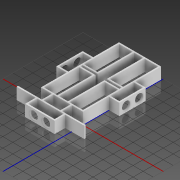
# Autodesk Inventor part: Motorcompartiment
Saved by Autodesk Inventor 2020.2 (Build 242310000, 310)
## iProperties
Created: 2019-12-09
Part Number: Motorcompartiment
Material: Generic
Document SubType Name: Modeling
Designer: Berkant
Density: 1 g/cm^3
Appearance: Default
Author: Berkant
Autodesk Inventor part; units mm, degrees
ref_plane "YZ Plane" through (0, 0, 0) normal (1, 0, 0) x (0, 1, 0)
ref_plane "XZ Plane" through (0, 0, 0) normal (0, 1, 0) x (-1, 0, 0)
ref_plane "XY Plane" through (0, 0, 0) normal (0, 0, 1) x (1, 0, 0)
sketch "Sketch1" plane through (0, 0, 0) normal (0, 1, 0) x (-1, 0, 0)
  line L0 (0, 0) -> (84, 0)
  line L1 (84, 0) -> (84, -156)
  line L2 (0, -156) -> (0, 0)
  line L3 (0, 0) -> (3, 0) construction
  line L4 (3, 0) -> (3, -3) construction
  line L5 (3, -3) -> (0, -3) construction
  line L6 (0, -3) -> (0, 0) construction
  line L7 (84, -153) -> (84, -156) construction
  line L8 (3, -3) -> (30, -3)
  line L9 (30, -3) -> (30, -73)
  line L10 (30, -73) -> (3, -73)
  line L11 (3, -73) -> (3, -3)
  line L12 (78, -153) -> (54, -153)
  line L13 (54, -153) -> (54, -83)
  line L14 (54, -83) -> (81, -83)
  line L15 (81, -83) -> (81, -153)
  line L16 (0, -153) -> (0, -156) construction
  line L17 (84, 0) -> (81, 0) construction
  line L18 (81, 0) -> (81, -3) construction
  line L19 (81, -3) -> (84, -3) construction
  line L20 (84, -3) -> (84, 0) construction
  line L21 (81, -3) -> (54, -3)
  line L22 (54, -3) -> (54, -73)
  line L23 (54, -73) -> (81, -73)
  line L24 (81, -73) -> (81, -3)
  line L25 (6, -153) -> (30, -153)
  line L26 (30, -153) -> (30, -83)
  line L27 (30, -83) -> (3, -83)
  line L28 (3, -83) -> (3, -153)
  line L29 (30, -3) -> (33, -3) construction
  line L30 (54, -153) -> (51, -153) construction
  line L31 (33, -3) -> (51, -3)
  line L32 (51, -153) -> (33, -153)
  line L33 (3, -73) -> (3, -76) construction
  line L34 (81, -83) -> (81, -80) construction
  line L35 (81, -76) -> (81, -80)
  line L36 (3, -80) -> (3, -76)
  line L37 (33, -153) -> (33, -80)
  line L38 (33, -76) -> (33, -3)
  line L39 (3, -76) -> (33, -76)
  line L40 (51, -76) -> (81, -76)
  line L41 (81, -80) -> (51, -80)
  line L42 (33, -80) -> (3, -80)
  line L43 (51, -3) -> (51, -76)
  line L44 (51, -80) -> (51, -153)
  line L45 (6, -153) -> (78, -153)
  line L46 (3, -153) -> (6, -153)
  line L47 (6, -156) -> (3, -156)
  line L48 (81, -153) -> (78, -153)
  line L49 (78, -156) -> (81, -156)
  line L50 (6, -156) -> (78, -156)
  line L51 (81, -156) -> (84, -156)
  line L52 (3, -156) -> (0, -156)
  dimension "d1" = 156
  dimension "d12" = 3
  dimension "d13" = 3
  dimension "d15" = 70
  dimension "d17" = 70
  dimension "d66" = 3
  dimension "d68" = 3
  constraints: 106 end point, 25 parallel, 16 horizontal, 11 perpendicular, 2 vertical, 1 collinear
  measures "d1" distance of L0.end L1.end
  measures "d12" distance of L19.end L18.end
  measures "d13" distance of L18.end L17.end
  measures "d15" distance of L22.end L21.end
  measures "d17" distance of L26.end L25.end
  measures "d66" distance of L25.start L47.start
  measures "d68" distance of L12.start L49.start
extrude "Extrusion1" add sketch "Sketch1" along normal blind 23
sketch "Sketch5" plane through (0, 0, 0) normal (1, 0, 0) x (0, 0, -1)
  circle A0 centre (16.6, 11.5) radius 3.5 projected
  circle A1 centre (139.4, 11.5) radius 3.5 projected
  line L0 (153, 23) -> (83, 23) projected
  line L1 (156, 0) -> (0, 0) projected
  line L2 (16.6, 11.5) -> (51.6, 11.5)
  line L3 (139.4, 11.5) -> (104.4, 11.5)
  line L4 (51.6, 23) -> (104.4, 23)
  line L5 (104.4, 23) -> (104.4, 0)
  line L6 (104.4, 0) -> (51.6, 0)
  line L7 (51.6, 0) -> (51.6, 23)
  point P0 (162, 0)
  dimension "d97" = 35
  dimension "d98" = 35
  constraints: 12 end point, 3 horizontal, 2 parallel, 1 perpendicular, 1 point on line
  measures "d97" distance of L2.start L2.end
  measures "d98" distance of L3.start L3.end
extrude "Extrusion6" add sketch "Sketch5" along normal blind 21 contours L5 L1 L7 L4 L0
sketch "Sketch6" plane through (0, 23, 0) normal (0, 1, 0) x (1, 0, 0)
  line L0 (0, 51.6) -> (21, 51.6) projected
  line L1 (21, 51.6) -> (18, 51.6)
  line L2 (18, 51.6) -> (18, 54.6)
  line L3 (18, 54.6) -> (21, 54.6)
  line L4 (21, 54.6) -> (21, 51.6)
  line L5 (0, 104.4) -> (21, 104.4) projected
  line L6 (21, 104.4) -> (18, 104.4)
  line L7 (18, 104.4) -> (18, 101.4)
  line L8 (18, 101.4) -> (21, 101.4)
  line L9 (21, 101.4) -> (21, 104.4)
  line L10 (18, 54.6) -> (0, 54.6)
  line L11 (18, 54.6) -> (18, 101.4)
  line L12 (18, 101.4) -> (0, 101.4)
  line L13 (0, 54.6) -> (0, 101.4)
  line L14 (-84, 156) -> (-84, 0) projected
  line L15 (-84, 54.6) -> (-102, 54.6)
  line L16 (-84, 54.6) -> (-66, 54.6) construction
  line L17 (-102, 54.6) -> (-102, 101.4)
  line L18 (-102, 101.4) -> (-84, 101.4)
  line L19 (-84, 101.4) -> (-84, 104.4)
  line L20 (-84, 104.4) -> (-105, 104.4)
  line L21 (-105, 104.4) -> (-105, 51.6)
  line L22 (-105, 51.6) -> (-84, 51.6)
  line L23 (-84, 51.6) -> (-84, 54.6)
  point P0 (0, 0)
  point P1 (21, 49.6)
  point P2 (21, 106.4)
  dimension "d99" = 3
  dimension "d100" = 3
  dimension "d101" = 3
  dimension "d102" = 3
  dimension "d112" = 18
  dimension "d113" = 180
  dimension "d114" = 3
  dimension "d115" = 21
  constraints: 42 end point, 8 perpendicular, 6 horizontal, 4 parallel, 3 point on line, 2 vertical, 1 collinear
  measures "d99" distance of L2.end L3.end
  measures "d100" distance of L1.end L2.end
  measures "d101" distance of L8.end L7.end
  measures "d102" distance of L7.end L6.end
  measures "d112" distance of L15.start L15.end
  measures "d113" angle of L15 L16
  measures "d114" distance of L18.end L19.end
  measures "d115" distance of L19.end L20.end
extrude "Extrusion7" cut sketch "Sketch6" against normal up to surface (23 mm away) contours L10 L13 L12 L11
extrude "Extrusion10" add sketch "Sketch6" against normal up to surface (23 mm away) contours L14 L18 L17 L15 L22 L21 L20
sketch "Sketch7" plane through (21, 0, 0) normal (1, 0, 0) x (0, 0, -1)
  line L0 (51.6, 0) -> (104.4, 0) projected
  circle A0 centre (91, 11.5) radius 8
  circle A1 centre (65, 11.5) radius 8
  line L1 (104.4, 23) -> (104.4, 0) projected
  line L2 (104.4, 23) -> (91, 23)
  line L3 (91, 23) -> (91, 11.5)
  line L4 (91, 11.5) -> (104.4, 11.5)
  line L5 (104.4, 11.5) -> (104.4, 23)
  circle A2 centre (91, 11.5) radius 8
  circle A3 centre (65, 11.5) radius 8
  point P0 (0, 0)
  dimension "d108" = 16
  dimension "d109" = 16
  dimension "d118" = 13.4
  dimension "d119" = 11.5
  constraints: 8 end point, 4 centre point, 2 coincident, 2 concentric, 2 parallel, 1 horizontal, 1 perpendicular
  measures "d108" diameter of A0
  measures "d109" diameter of A1
  measures "d118" distance of L4.end L3.end
  measures "d119" distance of L3.end L2.end
extrude "Extrusion9" cut sketch "Sketch7" against normal up to surface (3 mm away) contours L4 L3 A0 | A0 L3 L4 | A1
sketch "Sketch9" plane through (-105, 23, -104.4) normal (-1, 0, 0) x (0, 0, 1)
  line L0 (0, 0) -> (0, -23) projected
  line L1 (0, 0) -> (13.4, 0)
  line L2 (13.4, 0) -> (13.4, -11.5)
  line L3 (13.4, -11.5) -> (0, -11.5)
  line L4 (0, -11.5) -> (0, 0)
  circle A0 centre (13.4, -11.5) radius 8
  line L5 (0, 0) -> (52.8, 0) projected
  line L6 (52.8, 0) -> (39.4, 0)
  line L7 (39.4, 0) -> (39.4, -11.5)
  line L8 (39.4, -11.5) -> (52.8, -11.5)
  line L9 (52.8, -11.5) -> (52.8, 0)
  circle A1 centre (39.4, -11.5) radius 8
  point P0 (104.4, -23)
  dimension "d120" = 13.4
  dimension "d121" = 11.5
  dimension "d122" = 16
  dimension "d123" = 13.4
  dimension "d124" = 11.5
  dimension "d125" = 16
  constraints: 16 end point, 4 parallel, 2 centre point, 2 coincident, 2 horizontal, 2 perpendicular
  measures "d120" distance of L2.end L3.end
  measures "d121" distance of L1.end L2.end
  measures "d122" diameter of A0
  measures "d123" distance of L8.end L7.end
  measures "d124" distance of L7.end L6.end
  measures "d125" diameter of A1
extrude "Extrusion11" cut sketch "Sketch9" against normal blind 10 contours A0 L2 L3 | L3 L2 A0 | A1 L8 L7 | L7 L8 A1
sketch "Sketch10" plane through (-84, 0, 0) normal (0, 0, 1) x (1, 0, 0)
  line L0 (25, 23) -> (25, 0)
  line L1 (0, 0) -> (84, 0) projected
  line L2 (25, 0) -> (22, 0)
  line L3 (22, 0) -> (22, 23)
  line L4 (22, 23) -> (25, 23)
  line L5 (59, 23) -> (59, 0)
  line L6 (81, 0) -> (54, 0) projected
  line L7 (59, 0) -> (62, 0)
  line L8 (62, 0) -> (62, 23)
  line L9 (62, 23) -> (59, 23)
  point P0 (0, 23)
  point P1 (84, 23)
  dimension "d128" = 25
  dimension "d129" = 3
  dimension "d130" = 25
  dimension "d131" = 3
  constraints: 16 end point, 4 point on line, 2 horizontal, 1 perpendicular
  measures "d128" distance of point (0, 23) L0.start
  measures "d129" distance of L0.end L2.end
  measures "d130" distance of point (84, 23) L5.start
  measures "d131" distance of L5.end L7.end
extrude "Extrusion12" add sketch "Sketch10" along normal blind 23
sketch "Sketch11" plane through (-62, 0, 0) normal (-1, 0, 0) x (0, 0, 1)
  line L0 (0, 0) -> (23, 0) projected
  line L1 (23, 23) -> (20, 23)
  line L2 (20, 23) -> (20, 0)
  line L3 (20, 0) -> (23, 0)
  line L4 (23, 0) -> (23, 23)
  dimension "d134" = 3
  constraints: 8 end point, 2 parallel, 1 horizontal, 1 perpendicular, 1 point on line
  measures "d134" distance of L3.end L2.end
extrude "Extrusion13" add sketch "Sketch11" along normal blind 47.5 and the other way blind 87.5
sketch "Sketch12" plane through (-84, 0, 23) normal (0, 0, 1) x (1, 0, 0)
  line L0 (109.5, 23) -> (62, 23) projected
  line L1 (109.5, 23) -> (71.4, 23)
  line L2 (71.4, 23) -> (71.4, 0)
  line L3 (-25.5, 0) -> (109.5, 0) projected
  line L4 (109.5, 0) -> (62, 0) projected
  line L5 (71.4, 23) -> (68.4, 23)
  line L6 (68.4, 23) -> (68.4, 0)
  line L7 (68.4, 0) -> (71.4, 0)
  line L8 (71.4, 0) -> (71.4, 23)
  line L9 (12.6, 23) -> (12.6, 0)
  line L10 (22, 0) -> (-25.5, 0) projected
  line L11 (12.6, 23) -> (15.6, 23)
  line L12 (15.6, 23) -> (15.6, 0)
  line L13 (15.6, 0) -> (12.6, 0)
  line L14 (12.6, 0) -> (12.6, 23)
  point P0 (84, 0)
  point P1 (-25.5, 23)
  point P2 (15.6, 0)
  dimension "d139" = 38.1
  dimension "d140" = 3
  dimension "d141" = 38.1
  dimension "d142" = 3
  constraints: 22 end point, 4 parallel, 4 perpendicular, 4 point on line, 3 horizontal
  measures "d139" distance of L0.start L1.end
  measures "d140" distance of L7.end L6.end
  measures "d141" distance of point (-25.5, 23) L9.start
  measures "d142" distance of L12.end L13.end
extrude "Extrusion14" add sketch "Sketch12" along normal blind 21
sketch "Sketch13" plane through (-71.4, 0, 23) normal (-1, 0, 0) x (0, 0, 1)
  line L0 (0, 23) -> (21, 23) projected
  line L1 (0, 0) -> (21, 0) projected
  line L2 (21, 23) -> (18, 23)
  line L3 (18, 23) -> (18, 0)
  line L4 (18, 0) -> (21, 0)
  line L5 (21, 0) -> (21, 23)
  point P0 (-23, 0)
  point P1 (18, 23)
  dimension "d145" = 3
  constraints: 8 end point, 2 parallel, 1 horizontal, 1 perpendicular, 1 point on line
  measures "d145" distance of L4.end L3.end
extrude "Extrusion15" add sketch "Sketch13" against normal up to surface (58.8 mm away)
sketch "Sketch14" plane through (-84, 0, 44) normal (0, 0, 1) x (1, 0, 0)
  line L0 (71.4, 23) -> (54.4, 23)
  line L1 (54.4, 23) -> (54.4, 11.5)
  line L2 (54.4, 11.5) -> (71.4, 11.5)
  line L3 (71.4, 11.5) -> (71.4, 23)
  circle A0 centre (54.4, 11.5) radius 8
  line L4 (71.4, 23) -> (12.6, 23) projected
  line L5 (12.6, 23) -> (29.6, 23)
  line L6 (29.6, 23) -> (29.6, 11.5)
  line L7 (29.6, 11.5) -> (12.6, 11.5)
  line L8 (12.6, 11.5) -> (12.6, 23)
  circle A1 centre (29.6, 11.5) radius 8
  point P0 (84, 0)
  dimension "d148" = 17
  dimension "d149" = 11.5
  dimension "d150" = 16
  dimension "d151" = 17
  dimension "d152" = 11.5
  dimension "d153" = 16
  constraints: 16 end point, 4 parallel, 2 centre point, 2 coincident, 2 horizontal, 2 perpendicular
  measures "d148" distance of L2.end L1.end
  measures "d149" distance of L1.end L0.end
  measures "d150" diameter of A0
  measures "d151" distance of L6.end L7.end
  measures "d152" distance of L5.end L6.end
  measures "d153" diameter of A1
extrude "Extrusion16" cut sketch "Sketch14" against normal blind 10 contours A0 L2 L1 | L1 L2 A0 | A1 L7 L6 | L6 L7 A1
body "Solid1"
